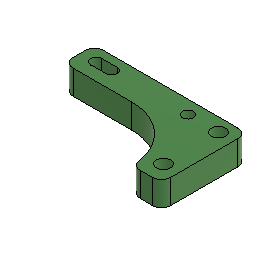
3d touch bracket v3 (Autodesk Fusion 360 design; units mm, degrees)
Autodesk Fusion 360 part; units mm, degrees
sketch "Sketch1" plane through (0, 0, 0) normal (0, 0, 1) x (1, 0, 0)
  line L0 (0, 0) -> (50, 0)
  line L1 (50, 0) -> (50, 10)
  line L2 (50, 10) -> (0, 10)
  line L3 (0, 10) -> (0, 0)
  line L4 (50, 0) -> (40, 0)
  line L5 (40, 0) -> (40, -18)
  line L6 (40, -18) -> (50, -18)
  line L7 (50, -18) -> (50, 0)
  circle A0 centre (5, 5.625) radius 1.8
  circle A1 centre (35, 5.625) radius 1.8
  circle A2 centre (45, 5.625) radius 2.3
  circle A3 centre (45, -12.375) radius 2.3
  circle A4 centre (10, 5.625) radius 1.8
  line L8 (5.039, 3.8254) -> (10, 3.8254)
  line L9 (10, 7.425) -> (5, 7.425)
  dimension "d1" = 50
  dimension "d2" = 10
  dimension "d3" = 10
  dimension "d4" = 18
  dimension "d5" = 3.6
  dimension "d6" = 3.6
  dimension "d7" = 5
  dimension "d8" = 30
  dimension "d9" = 4.6
  dimension "d10" = 10
  dimension "d11" = 4.6
  dimension "d12" = 18
  dimension "d20" = 3.6
  dimension "d21" = 5.625
  dimension "d22" = 5
  constraint horizontal L0
  constraint vertical L1
  constraint horizontal L2
  constraint vertical L3
  constraint coincident L0.start L3.end
  constraint horizontal L4
  constraint vertical L5
  constraint horizontal L6
  constraint vertical L7
  constraint horizontal A0.centre A1.centre
  constraint horizontal A0.centre A4.centre
  constraint horizontal A1.centre A2.centre
  constraint vertical A2.centre A3.centre
  constraint coincident A0 L8.start
  constraint horizontal L8
  constraint coincident A4 L9.start
  constraint coincident A0 L9.end
  constraint tangent A0 L9
  constraint parallel L8 L9
  measures "d1" distance of L0.start L0.end
  measures "d2" distance of L0.start L2.end
  measures "d3" distance of L0.end L4.end
  measures "d4" distance of L0.end L6.end
  measures "d5" diameter of A0
  measures "d6" diameter of A1
  measures "d7" distance of L3 A0.centre
  measures "d8" distance of A0.centre A1.centre
  measures "d9" diameter of A2
  measures "d10" distance of A1.centre A2.centre
  measures "d11" diameter of A3
  measures "d12" distance of A2.centre A3.centre
  measures "d20" diameter of A4
  measures "d21" distance of L0 A0.centre
  measures "d22" distance of A0.centre A4.centre
extrude "Extrude1" add sketch "Sketch1" along normal blind 8
fillet "Fillet1" radius 3 5 edges at (40, -18, 4) (50, -18, 4) (0, 0, 4) (50, 10, 4) (0, 10, 4)
fillet "Fillet2" radius 18 1 edges at (40, 0, 4)
chamfer "Chamfer1" [suppressed]
equation "d4 = d12"
equation "d6 = d5"
equation "d9 = d11"
equation "d20 = d5"
equation "d21 = 9 / 16 * d2"
